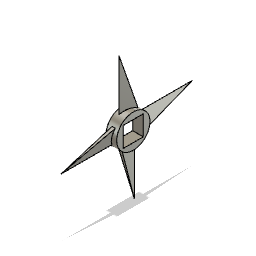
Ninja_Star v2 (Autodesk Fusion 360 design; units mm, degrees)
Autodesk Fusion 360 part; units mm, degrees
sketch "Sketch1" plane through (0, 0, 0) normal (1, 0, 0) x (0, 0, -1)
  circle A0 centre (0, 0) radius 12.5
  line L0 (7.5, 7.5) -> (-7.5, 7.5)
  line L1 (-7.5, 7.5) -> (-7.5, -7.5)
  line L2 (-7.5, -7.5) -> (7.5, -7.5)
  line L3 (7.5, -7.5) -> (7.5, 7.5)
  line L4 (7.5, 7.5) -> (-7.5, -7.5) construction
  line L5 (-7.5, 7.5) -> (7.5, -7.5) construction
  dimension "d1" = 25
  dimension "d2" = 15
  dimension "d3" = 15
  constraint coincident A0.centre origin
  constraint horizontal L0
  constraint perpendicular L0 L1
  constraint parallel L0 L2
  constraint parallel L1 L3
  constraint coincident L4 A0.centre
  constraint coincident L5 A0.centre
  measures "d1" diameter of A0
  measures "d2" distance of L1.end L2.end
  measures "d3" distance of L0.end L1.end
extrude "Extrude1" add sketch "Sketch1" along normal blind 8
sketch "Sketch2" plane through (0, 0, 0) normal (0, 1, 0) x (1, 0, 0)
sketch "Sketch3" plane through (8, 0, 0) normal (1, 0, 0) x (0, 0, -1)
  line L0 (7.5, 7.5) -> (7.5, -7.5)
  line L1 (7.5, -7.5) -> (-7.5, -7.5)
  line L2 (-7.5, -7.5) -> (-7.5, 7.5)
  line L3 (-7.5, 7.5) -> (7.5, 7.5)
  circle A0 centre (0, 0) radius 12.5
  line L4 (-5.7956, 9.4779) -> (6.4844, 9.4779)
  line L5 (6.4844, 9.4779) -> (-5.7956, 49.4779)
  line L6 (-5.7956, 49.4779) -> (-5.7956, 9.4779)
  dimension "d14" = 40
  constraint perpendicular L0 L4
  constraint perpendicular L4 L6
  measures "d14" distance of L4.start L5.end
extrude "Extrude2" add sketch "Sketch3" along normal blind 2.5 from surface at -5 contours A0 L5 L6
sketch "Sketch4" plane through (0, 0, 0) normal (0, 1, 0) x (1, 0, 0)
  line L0 (2.9867, -5.8624) -> (5.5, -5.8624)
  line L1 (5.5, -5.8624) -> (5.5, 6)
  line L2 (5.5, 6) -> (2.9867, -5.8624)
  constraint horizontal L0
  constraint perpendicular L0 L1
extrude "Extrude3" cut sketch "Sketch4" against normal blind 39 from surface at 50
pattern_circular "C-Pattern1" count 4 over 360 about axis through (1.75, 0, 0) along (1, 0, 0) of "Extrude2", "Extrude3"
sketch "Sketch5" plane through (0, 0, 0) normal (0, 1, 0) x (-1, 0, 0)
sketch "Sketch6" plane through (8, 0, 0) normal (1, 0, 0) x (0, 0, -1)
  line L0 (7.5, 7.5) -> (7.5, -7.5)
  line L1 (7.5, -7.5) -> (-7.5, -7.5)
  line L2 (-7.5, -7.5) -> (-7.5, 7.5)
  line L3 (-7.5, 7.5) -> (7.5, 7.5)
  circle A0 centre (0, 0) radius 12.5
  circle A1 centre (0, 0) radius 12.5
  line L4 (7.5, 7.5) -> (-7.5, 7.5)
  line L5 (-7.5, 7.5) -> (-7.5, -7.5)
  line L6 (-7.5, -7.5) -> (7.5, -7.5)
  line L7 (7.5, -7.5) -> (7.5, 7.5)
  line L8 (7.5, 7.5) -> (-7.5, -7.5) construction
  line L9 (-7.5, 7.5) -> (7.5, -7.5) construction
  constraint coincident A0.centre A1.centre
  constraint horizontal L4
  constraint perpendicular L4 L5
  constraint parallel L4 L6
  constraint parallel L5 L7
  constraint coincident L0.start L3.end
  constraint coincident L8 A0.centre
  constraint coincident L9 A0.centre
extrude "Extrude4" add sketch "Sketch6" against normal blind 8
